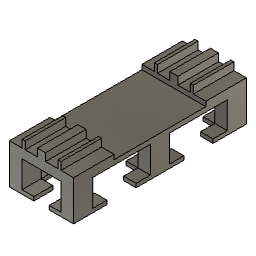
cell and oil channel flow sensors holder v5 kanishk fused v2 (Autodesk Fusion 360 design; units mm, degrees)
Autodesk Fusion 360 part; units mm, degrees
note: some values were not read from the file. Chosen so that the rebuilt part matches the saved one: which bodies a step acts on; which face or edge a step refers to.
sketch "Sketch1" plane through (0, 0, 0) normal (0, 0, 1) x (1, 0, 0)
  line L0 (0, 0) -> (86.6, 0)
  line L1 (86.6, 0) -> (86.6, 120)
  line L2 (86.6, 120) -> (0, 120)
  line L3 (0, 120) -> (0, 0)
  line L4 (43.3, 120) -> (35, 120)
  line L5 (35, 120) -> (35, 0)
  line L6 (35, 0) -> (43.3, 0)
  line L7 (43.3, 0) -> (43.3, 120)
  line L8 (43.3, 120) -> (51.6, 120)
  line L9 (51.6, 120) -> (51.6, 0)
  line L10 (51.6, 0) -> (43.3, 0)
  line L11 (43.3, 0) -> (43.3, 120)
  line L12 (51.6, 120) -> (66.2, 120)
  line L13 (66.2, 120) -> (66.2, 0)
  line L14 (66.2, 0) -> (51.6, 0)
  line L15 (51.6, 0) -> (51.6, 120)
  line L16 (66.2, 120) -> (70.2, 120)
  line L17 (70.2, 120) -> (70.2, 0)
  line L18 (70.2, 0) -> (66.2, 0)
  line L19 (66.2, 0) -> (66.2, 120)
  line L20 (70.2, 120) -> (84.8, 120)
  line L21 (84.8, 120) -> (84.8, 0)
  line L22 (84.8, 0) -> (70.2, 0)
  line L23 (70.2, 0) -> (70.2, 120)
  line L24 (84.8, 120) -> (90.8, 120)
  line L25 (90.8, 120) -> (90.8, 0)
  line L26 (90.8, 0) -> (84.8, 0)
  line L27 (84.8, 0) -> (84.8, 120)
  line L28 (35, 120) -> (20.4, 120)
  line L29 (20.4, 120) -> (20.4, 0)
  line L30 (20.4, 0) -> (35, 0)
  line L31 (35, 0) -> (35, 120)
  line L32 (20.4, 120) -> (16.4, 120)
  line L33 (16.4, 120) -> (16.4, 0)
  line L34 (16.4, 0) -> (20.4, 0)
  line L35 (20.4, 0) -> (20.4, 120)
  line L36 (16.4, 120) -> (1.8, 120)
  line L37 (1.8, 120) -> (1.8, 0)
  line L38 (1.8, 0) -> (16.4, 0)
  line L39 (16.4, 0) -> (16.4, 120)
  line L40 (1.8, 120) -> (-4.2, 120)
  line L41 (-4.2, 120) -> (-4.2, 0)
  line L42 (-4.2, 0) -> (1.8, 0)
  line L43 (1.8, 0) -> (1.8, 120)
  dimension "d1" = 86.6
  dimension "d2" = 120
  dimension "d3" = 8.3
  dimension "d4" = 120
  dimension "d5" = 8.3
  dimension "d6" = 120
  dimension "d7" = 14.6
  dimension "d8" = 120
  dimension "d9" = 4
  dimension "d10" = 120
  dimension "d11" = 14.6
  dimension "d12" = 120
  dimension "d13" = 6
  dimension "d14" = 14.6
  dimension "d15" = 120
  dimension "d16" = 4
  dimension "d17" = 120
  dimension "d18" = 14.6
  dimension "d19" = 120
  dimension "d20" = 6
  dimension "d21" = 120
  constraint horizontal L0
  constraint vertical L1
  constraint horizontal L2
  constraint vertical L3
  constraint coincident L0.start L3.end
  constraint horizontal L4
  constraint vertical L5
  constraint horizontal L6
  constraint vertical L7
  constraint midpoint L2 L4.start
  constraint horizontal L8
  constraint vertical L9
  constraint horizontal L10
  constraint vertical L11
  constraint horizontal L12
  constraint vertical L13
  constraint horizontal L14
  constraint vertical L15
  constraint horizontal L16
  constraint vertical L17
  constraint horizontal L18
  constraint vertical L19
  constraint horizontal L20
  constraint vertical L21
  constraint horizontal L22
  constraint vertical L23
  constraint horizontal L24
  constraint vertical L25
  constraint horizontal L26
  constraint vertical L27
  constraint horizontal L28
  constraint vertical L29
  constraint horizontal L30
  constraint vertical L31
  constraint horizontal L32
  constraint vertical L33
  constraint horizontal L34
  constraint vertical L35
  constraint horizontal L36
  constraint vertical L37
  constraint horizontal L38
  constraint vertical L39
  constraint horizontal L40
  constraint vertical L41
  constraint horizontal L42
  constraint vertical L43
  measures "d1" distance of L0.start L0.end
  measures "d2" distance of L0.start L2.end
  measures "d3" distance of L4.start L4.end
  measures "d4" distance of L4.start L6.end
  measures "d5" distance of L4.start L8.end
  measures "d6" distance of L4.start L6.end
  measures "d7" distance of L8.end L12.end
  measures "d8" distance of L8.end L9.end
  measures "d9" distance of L12.end L16.end
  measures "d10" distance of L12.end L13.end
  measures "d11" distance of L16.end L20.end
  measures "d12" distance of L16.end L17.end
  measures "d13" distance of L20.end L24.end
  measures "d14" distance of L4.end L28.end
  measures "d15" distance of L4.end L5.end
  measures "d16" distance of L28.end L32.end
  measures "d17" distance of L28.end L29.end
  measures "d18" distance of L32.end L36.end
  measures "d19" distance of L32.end L33.end
  measures "d20" distance of L36.end L40.end
  measures "d21" distance of L36.end L37.end
extrude "Extrude1" add sketch "Sketch1" along normal blind 52.3 contours L0 L2 L3 L37 L40 L42 L43 | L0 L2 L33 L36 L37 L38 L39 L43 | L0 L2 L29 L32 L33 L34 L35 L39 | L0 L2 L5 L28 L29 L30 L31 L35 | L0 L2 L4 L5 L6 L7 L11 L31 | L0 L2 L7 L8 L9 L10 L11 L15 | L0 L2 L9 L12 L13 L14 L15 L19 | L0 L2 L13 L16 L17 L18 L19 L23 | L0 L2 L17 L20 L21 L22 L23 L27 | L0 L1 L2 L21 L24 L26 L27 makes body 1
extrude "Extrude2" add sketch "Sketch1" along normal blind 62.3 contours L0 L2 L4 L5 L6 L7 L11 L31 | L0 L2 L7 L8 L9 L10 L11 L15 bodies 1
extrude "Extrude3" add sketch "Sketch1" along normal blind 62.3 contours L0 L2 L3 L37 L40 L42 L43 | L3 L40 L41 L42 | L0 L2 L29 L32 L33 L34 L35 L39 | L0 L2 L13 L16 L17 L18 L19 L23 | L0 L1 L2 L21 L24 L26 L27 | L1 L24 L25 L26 bodies 1
extrude "Extrude4" cut sketch "Sketch1" along normal blind 37.3 contours L3 L40 L41 L42 | L1 L24 L25 L26 bodies 1
sketch "Sketch2" plane through (0, 0, 0) normal (0, -1, 0) x (1, 0, 0)
  line L0 (86.6, 37.3) -> (90.8, 37.3)
  line L1 (90.8, 37.3) -> (90.8, 62.3)
  line L2 (90.8, 62.3) -> (84.8, 62.3)
  line L3 (84.8, 62.3) -> (84.8, 52.3)
  line L4 (84.8, 52.3) -> (70.2, 52.3)
  line L5 (70.2, 52.3) -> (70.2, 62.3)
  line L6 (70.2, 62.3) -> (66.2, 62.3)
  line L7 (66.2, 62.3) -> (66.2, 52.3)
  line L8 (66.2, 52.3) -> (51.6, 52.3)
  line L9 (51.6, 52.3) -> (51.6, 62.3)
  line L10 (51.6, 62.3) -> (35, 62.3)
  line L11 (35, 62.3) -> (35, 52.3)
  line L12 (35, 52.3) -> (20.4, 52.3)
  line L13 (20.4, 52.3) -> (20.4, 62.3)
  line L14 (20.4, 62.3) -> (16.4, 62.3)
  line L15 (16.4, 62.3) -> (16.4, 52.3)
  line L16 (16.4, 52.3) -> (1.8, 52.3)
  line L17 (1.8, 52.3) -> (1.8, 62.3)
  line L18 (1.8, 62.3) -> (-4.2, 62.3)
  line L19 (-4.2, 62.3) -> (-4.2, 37.3)
  line L20 (-4.2, 37.3) -> (0, 37.3)
  line L21 (0, 37.3) -> (0, 0)
  line L22 (0, 0) -> (86.6, 0)
  line L23 (86.6, 0) -> (86.6, 37.3)
  line L24 (0, 0) -> (10, 0)
  line L25 (10, 0) -> (10, 10)
  line L26 (10, 10) -> (0, 10)
  line L27 (0, 10) -> (0, 0)
  line L28 (86.6, 0) -> (76.6, 0)
  line L29 (76.6, 0) -> (76.6, 10)
  line L30 (76.6, 10) -> (86.6, 10)
  line L31 (86.6, 10) -> (86.6, 0)
  line L32 (0, 15) -> (10, 15)
  line L33 (10, 15) -> (10, 25)
  line L34 (10, 25) -> (0, 25)
  line L35 (0, 25) -> (0, 15)
  line L36 (0, 30) -> (10, 30)
  line L37 (10, 30) -> (10, 40)
  line L38 (10, 40) -> (0, 40)
  line L39 (0, 40) -> (0, 30)
  line L40 (86.6, 14.8875) -> (76.6, 14.8875)
  line L41 (76.6, 14.8875) -> (76.6, 24.8875)
  line L42 (76.6, 24.8875) -> (86.6, 24.8875)
  line L43 (86.6, 24.8875) -> (86.6, 14.8875)
  line L44 (86.6, 30.0734) -> (76.6, 30.0734)
  line L45 (76.6, 30.0734) -> (76.6, 40.0734)
  line L46 (76.6, 40.0734) -> (86.6, 40.0734)
  line L47 (86.6, 40.0734) -> (86.6, 30.0734)
  dimension "d30" = 10
  dimension "d31" = 10
  dimension "d32" = 10
  dimension "d33" = 10
  dimension "d34" = 10
  dimension "d35" = 10
  dimension "d36" = 10
  dimension "d37" = 10
  dimension "d38" = 10
  dimension "d39" = 10
  dimension "d40" = 10
  dimension "d41" = 10
  constraint horizontal L24
  constraint vertical L25
  constraint horizontal L26
  constraint vertical L27
  constraint coincident L21.end L22.start
  constraint horizontal L28
  constraint vertical L29
  constraint horizontal L30
  constraint vertical L31
  constraint coincident L22.end L23.start
  constraint horizontal L32
  constraint vertical L33
  constraint horizontal L34
  constraint vertical L35
  constraint coincident L21 L32.start
  constraint horizontal L36
  constraint vertical L37
  constraint horizontal L38
  constraint vertical L39
  constraint coincident L21 L36.start
  constraint horizontal L40
  constraint vertical L41
  constraint horizontal L42
  constraint vertical L43
  constraint coincident L23 L40.start
  constraint horizontal L44
  constraint vertical L45
  constraint horizontal L46
  constraint vertical L47
  constraint coincident L23 L44.start
  measures "d30" distance of L21.end L24.end
  measures "d31" distance of L21.end L26.end
  measures "d32" distance of L22.end L28.end
  measures "d33" distance of L22.end L30.end
  measures "d34" distance of L32.start L32.end
  measures "d35" distance of L32.start L34.end
  measures "d36" distance of L36.start L36.end
  measures "d37" distance of L36.start L38.end
  measures "d38" distance of L40.start L40.end
  measures "d39" distance of L40.start L42.end
  measures "d40" distance of L44.start L44.end
  measures "d41" distance of L44.start L46.end
extrude "Extrude5" cut sketch "Sketch2" against normal blind 20 contours L21 L22 L24 L25 L26 L27 bodies 1
extrude "Extrude6" add sketch "Sketch2" along normal blind 20 contours L22 L23 L28 L29 L30 L31 bodies 1
extrude "Extrude7" add sketch "Sketch2" along normal blind 20 contours L21 L32 L33 L34 L35 bodies 1
extrude "Extrude8" cut sketch "Sketch2" against normal blind 20 contours L23 L40 L41 L42 L43 bodies 1
extrude "Extrude9" cut sketch "Sketch2" against normal blind 20 contours L21 L36 L37 L38 L39 bodies 1
extrude "Extrude10" add sketch "Sketch2" along normal blind 20 contours L23 L44 L45 L46 L47 bodies 1
sketch "Sketch3" plane through (0, 0, 0) normal (0, -1, 0) x (1, 0, 0)
  line L0 (0, 0) -> (86.5609, 0)
  line L1 (43.2804, 0) -> (16.2804, 0)
  line L2 (16.2804, 0) -> (16.2804, 40)
  line L3 (16.2804, 40) -> (43.2804, 40)
  line L4 (43.2804, 40) -> (43.2804, 0)
  line L5 (43.2804, 0) -> (70.2804, 0)
  line L6 (70.2804, 0) -> (70.2804, 40)
  line L7 (70.2804, 40) -> (43.2804, 40)
  line L8 (43.2804, 40) -> (43.2804, 0)
  dimension "d54" = 27
  dimension "d55" = 40
  dimension "d56" = 27
  dimension "d57" = 40
  constraint coincident L0.start origin
  constraint horizontal L0
  constraint horizontal L1
  constraint vertical L2
  constraint horizontal L3
  constraint vertical L4
  constraint midpoint L0 L1.start
  constraint horizontal L5
  constraint vertical L6
  constraint horizontal L7
  constraint vertical L8
  measures "d54" distance of L1.start L1.end
  measures "d55" distance of L1.start L3.end
  measures "d56" distance of L1.start L5.end
  measures "d57" distance of L1.start L3.end
sketch "Sketch4" plane through (86.6, 0, 0) normal (1, 0, 0) x (0, 1, 0)
  line L0 (0, 24.8875) -> (20, 24.8875)
  line L1 (20, 24.8875) -> (20, 14.8875)
  line L2 (20, 14.8875) -> (0, 14.8875)
  line L3 (0, 14.8875) -> (0, 10)
  line L4 (0, 10) -> (-20, 10)
  line L5 (-20, 10) -> (-20, 0)
  line L6 (-20, 0) -> (120, 0)
  line L7 (120, 0) -> (120, 37.3)
  line L8 (120, 37.3) -> (0, 37.3)
  line L9 (0, 37.3) -> (0, 40.0734)
  line L10 (0, 40.0734) -> (-20, 40.0734)
  line L11 (-20, 40.0734) -> (-20, 30.0734)
  line L12 (-20, 30.0734) -> (0, 30.0734)
  line L13 (0, 30.0734) -> (0, 24.8875)
  line L14 (30, 0) -> (100, 0)
  line L15 (100, 0) -> (100, 35)
  line L16 (100, 35) -> (30, 35)
  line L17 (30, 35) -> (30, 0)
  dimension "d58" = 70
  dimension "d59" = 35
  constraint horizontal L14
  constraint vertical L15
  constraint horizontal L16
  constraint vertical L17
  constraint coincident L6 L14.start
  measures "d58" distance of L14.start L14.end
  measures "d59" distance of L14.start L16.end
extrude "Extrude11" cut sketch "Sketch3" against normal blind 130 bodies 1
extrude "Extrude12" cut sketch "Sketch4" against normal blind 100 contours L6 L14 L15 L16 L17 bodies 1
sketch "Sketch5" plane through (0, 0, 0) normal (0, -1, 0) x (1, 0, 0)
sketch "Sketch6" plane through (0, 0, 62.3) normal (0, 0, 1) x (-1, 0, 0)
  line L0 (-84.8, 0) -> (-90.8, 0)
  line L1 (-90.8, 0) -> (-90.8, -120)
  line L2 (-90.8, -120) -> (-84.8, -120)
  line L3 (-84.8, -120) -> (-84.8, 0)
  line L4 (-84.8, 0) -> (-86.3, 0)
  line L5 (-86.3, 0) -> (-86.3, -120)
  line L6 (-86.3, -120) -> (-84.8, -120)
  line L7 (-84.8, -120) -> (-84.8, 0)
  dimension "d64" = 1.5
  dimension "d65" = 120
  constraint horizontal L4
  constraint vertical L5
  constraint horizontal L6
  constraint vertical L7
  constraint coincident L0.start L3.end
  measures "d64" distance of L0.start L4.end
  measures "d65" distance of L0.start L2.end
sketch "Sketch7" plane through (0, 0, 62.3) normal (0, 0, 1) x (-1, 0, 0)
  line L0 (-1.8, 0) -> (-1.8, -120)
  line L1 (-1.8, -120) -> (4.2, -120)
  line L2 (4.2, -120) -> (4.2, 0)
  line L3 (4.2, 0) -> (-1.8, 0)
  line L4 (-1.8, -120) -> (-0.3, -120)
  line L5 (-0.3, -120) -> (-0.3, 0)
  line L6 (-0.3, 0) -> (-1.8, 0)
  line L7 (-1.8, 0) -> (-1.8, -120)
  dimension "d66" = 1.5
  dimension "d67" = 120
  constraint horizontal L4
  constraint vertical L5
  constraint horizontal L6
  constraint vertical L7
  constraint coincident L0.end L1.start
  measures "d66" distance of L0.end L4.end
  measures "d67" distance of L0.end L0.start
extrude "Extrude13" cut sketch "Sketch6" sketch "Sketch7" against normal blind 10 contours L0 L2 L3 L4 L5 L6 L7 of sketch 2 contours L0 L1 L3 L4 L5 L6 L7 bodies 1
sketch "Sketch8" plane through (0, 0, 62.3) normal (0, 0, 1) x (-1, 0, 0)
  line L0 (-51.6, 0) -> (-51.6, -120)
  line L1 (-51.6, -120) -> (-35, -120)
  line L2 (-35, -120) -> (-35, 0)
  line L3 (-35, 0) -> (-51.6, 0)
  line L4 (-35, -120) -> (-36.5, -120)
  line L5 (-36.5, -120) -> (-36.5, 0)
  line L6 (-36.5, 0) -> (-35, 0)
  line L7 (-35, 0) -> (-35, -120)
  line L8 (-51.6, -120) -> (-50.1, -120)
  line L9 (-50.1, -120) -> (-50.1, 0)
  line L10 (-50.1, 0) -> (-51.6, 0)
  line L11 (-51.6, 0) -> (-51.6, -120)
  dimension "d70" = 1.5
  dimension "d71" = 120
  dimension "d72" = 1.5
  dimension "d73" = 120
  constraint horizontal L4
  constraint vertical L5
  constraint horizontal L6
  constraint vertical L7
  constraint coincident L1.end L2.start
  constraint horizontal L8
  constraint vertical L9
  constraint horizontal L10
  constraint vertical L11
  constraint coincident L0.end L1.start
  measures "d70" distance of L1.end L4.end
  measures "d71" distance of L1.end L2.end
  measures "d72" distance of L0.end L8.end
  measures "d73" distance of L0.end L0.start
extrude "Extrude14" cut sketch "Sketch8" against normal blind 10 contours L0 L1 L3 L8 L9 L10 L11 | L1 L2 L3 L4 L5 L6 L7 bodies 1
extrude "Extrude15" cut sketch "Sketch1" along normal blind 100 contours L3 L40 L41 L42 | L1 L24 L25 L26 bodies 1
extrude "Extrude16" cut 1 faces at (86.4, 80, 62.3) along direction (0, 0, -1) blind 10 on bodies 1 bodies 1
extrude "Extrude17" cut 1 faces at (0.1, 80, 62.3) along direction (0, 0, -1) blind 10 on bodies 1 bodies 1
sketch "Sketch9" plane through (0, 0, 0) normal (0, -1, 0) x (1, 0, 0)
extrude "Extrude18" cut 3 faces at (3.3333, -20, 21.6667) (83.2667, -20, 33.4067) (83.2667, -20, 3.3333) along direction (0, 1, 0) blind 20 on bodies 1 bodies 1
extrude "Extrude19" add 1 faces at (76.6, 6.6667, 18.2208) along direction (1, 0, 0) blind 10 on bodies 1 bodies 1
extrude "Extrude20" add 2 faces at (3.3333, 20, 36.6667) (6.6667, 20, 3.3333) along direction (0, -1, 0) blind 20 on bodies 1 bodies 1
mirror "Mirror1" about plane through (51.6, 120, 0) normal (0, 1, 0) of bodies 1 merged
extrude "Extrude21" cut 1 faces at (81.1601, 240, 30.7667) along direction (0, -1, 0) blind 5 on bodies 1 bodies 1
extrude "Extrude22" cut 1 faces at (81.1601, 0, 30.7667) along direction (0, 1, 0) blind 5 on bodies 1 bodies 1
split "Split1" by plane through (36.5, 120, 62.3) normal (-1, 0, 0) bodies 1 makes body 2 at (0, 126.6667, 11.6667)
extrude "Extrude23" cut 2 faces at (36.5, 81.6667, 48.2) (36.5, 158.3333, 58.9667) along direction (1, 0, 0) blind 3 on bodies 1 bodies 1
move_body "Move1" bodies 2 to x (1, 0, 0) y (0, 1, 0) z (0, 0, 1) at (3, 0, 0)
combine "Combine1" operation add target body 1 tool bodies 2
sketch "Sketch10" plane through (19.2804, 0, 0) normal (1, 0, 0) x (0, 1, 0)
  line L0 (5, 40) -> (5, 0)
  line L1 (5, 0) -> (30, 0)
  line L2 (30, 0) -> (30, 35)
  line L3 (30, 35) -> (100, 35)
  line L4 (100, 35) -> (100, 0)
  line L5 (100, 0) -> (140, 0)
  line L6 (140, 0) -> (140, 35)
  line L7 (140, 35) -> (210, 35)
  line L8 (210, 35) -> (210, 0)
  line L9 (210, 0) -> (235, 0)
  line L10 (235, 0) -> (235, 40)
  line L11 (235, 40) -> (5, 40)
  line L12 (5, 0) -> (30, 0)
  line L13 (30, 0) -> (30, 5)
  line L14 (30, 5) -> (5, 5)
  line L15 (5, 5) -> (5, 0)
  line L16 (100, 0) -> (140, 0)
  line L17 (140, 0) -> (140, 5)
  line L18 (140, 5) -> (100, 5)
  line L19 (100, 5) -> (100, 0)
  line L20 (210, 0) -> (235, 0)
  line L21 (235, 0) -> (235, 5)
  line L22 (235, 5) -> (210, 5)
  line L23 (210, 5) -> (210, 0)
  line L24 (100, 35) -> (107.5, 35)
  line L25 (107.5, 35) -> (107.5, 0)
  line L26 (107.5, 0) -> (100, 0)
  line L27 (100, 0) -> (100, 35)
  line L28 (140, 0) -> (132.5, 0)
  line L29 (132.5, 0) -> (132.5, 35)
  line L30 (132.5, 35) -> (140, 35)
  line L31 (140, 35) -> (140, 0)
  dimension "d96" = 5
  dimension "d97" = 5
  dimension "d98" = 5
  dimension "d99" = 7.5
  dimension "d100" = 7.5
  dimension "d101" = 35
  constraint horizontal L12
  constraint vertical L13
  constraint horizontal L14
  constraint vertical L15
  constraint coincident L0.end L1.start
  constraint horizontal L16
  constraint vertical L17
  constraint horizontal L18
  constraint vertical L19
  constraint coincident L4.end L5.start
  constraint horizontal L20
  constraint vertical L21
  constraint horizontal L22
  constraint vertical L23
  constraint coincident L8.end L9.start
  constraint horizontal L24
  constraint vertical L25
  constraint horizontal L26
  constraint vertical L27
  constraint coincident L3.end L4.start
  constraint horizontal L28
  constraint vertical L29
  constraint horizontal L30
  constraint vertical L31
  constraint coincident L5.end L6.start
  measures "d96" distance of L0.end L14.end
  measures "d97" distance of L4.end L18.end
  measures "d98" distance of L8.end L22.end
  measures "d99" distance of L3.end L24.end
  measures "d100" distance of L5.end L28.end
  measures "d101" distance of L5.end L6.end
extrude "Extrude24" add sketch "Sketch10" along normal blind 51 contours L0 L1 L2 L12 L13 L14 L15 | L8 L9 L10 L20 L21 L22 L23 | L4 L5 L16 L18 L19 L25 L26 L27 | L5 L16 L18 L25 L29 | L5 L6 L16 L17 L18 L28 L29 L31 bodies 1
extrude "Extrude25" cut sketch "Sketch10" along normal blind 1000 and the other way blind 100 contours L4 L18 L24 L25 L27 | L4 L5 L16 L18 L19 L25 L26 L27 | L6 L18 L29 L30 L31 | L5 L6 L16 L17 L18 L28 L29 L31 bodies 1
sketch "Sketch12" plane through (0, 235, 0) normal (0, 1, 0) x (-1, 0, 0)
  line L0 (-86.6, 0) -> (-3, 0)
  line L1 (-3, 0) -> (-3, 52.3)
  line L2 (-3, 52.3) -> (-19.4, 52.3)
  line L3 (-19.4, 52.3) -> (-19.4, 62.3)
  line L4 (-19.4, 62.3) -> (-23.4, 62.3)
  line L5 (-23.4, 62.3) -> (-23.4, 52.3)
  line L6 (-23.4, 52.3) -> (-39.5, 52.3)
  line L7 (-39.5, 52.3) -> (-39.5, 62.3)
  line L8 (-39.5, 62.3) -> (-50.1, 62.3)
  line L9 (-50.1, 62.3) -> (-50.1, 52.3)
  line L10 (-50.1, 52.3) -> (-66.2, 52.3)
  line L11 (-66.2, 52.3) -> (-66.2, 62.3)
  line L12 (-66.2, 62.3) -> (-70.2, 62.3)
  line L13 (-70.2, 62.3) -> (-70.2, 52.3)
  line L14 (-70.2, 52.3) -> (-86.6, 52.3)
  line L15 (-86.6, 52.3) -> (-86.6, 0)
  line L16 (-19.2804, 5) -> (-70.2804, 5)
  line L17 (-70.2804, 5) -> (-70.2804, 40)
  line L18 (-70.2804, 40) -> (-19.2804, 40)
  line L19 (-19.2804, 40) -> (-19.2804, 5)
  line L20 (-70.2804, 5) -> (-86.6, 5)
  line L21 (-86.6, 5) -> (-86.6, 0)
  line L22 (-86.6, 0) -> (-70.2804, 0)
  line L23 (-70.2804, 0) -> (-70.2804, 5)
  line L24 (-19.2804, 5) -> (-3, 5)
  line L25 (-3, 5) -> (-3, 0)
  line L26 (-3, 0) -> (-19.2804, 0)
  line L27 (-19.2804, 0) -> (-19.2804, 5)
  line L28 (-44.8, 0) -> (-54.8, 0)
  line L29 (-54.8, 0) -> (-54.8, 5)
  line L30 (-54.8, 5) -> (-44.8, 5)
  line L31 (-44.8, 5) -> (-44.8, 0)
  line L32 (-34.8, 0) -> (-34.8, 5)
  dimension "d108" = 10
  constraint horizontal L20
  constraint vertical L21
  constraint horizontal L22
  constraint vertical L23
  constraint coincident L0.start L15.end
  constraint coincident L16.end L17.start
  constraint horizontal L24
  constraint vertical L25
  constraint horizontal L26
  constraint vertical L27
  constraint coincident L0.end L1.start
  constraint coincident L16.start L19.end
  constraint horizontal L28
  constraint vertical L29
  constraint horizontal L30
  constraint vertical L31
  constraint midpoint L0 L28.start
  constraint symmetric L28.end L31 L32.start
  constraint symmetric L29.end L31 L32.end
  measures "d108" distance of L28.start L28.end
extrude "Extrude26" cut sketch "Sketch12" against normal blind 1000 contours L0 L16 L28 L29 L30 L31 | L0 L16 L31 L32 bodies 1
extrude "Extrude27" add sketch "Sketch12" against normal blind 205 contours L0 L15 L20 L21 L22 L23 | L0 L1 L24 L25 L26 L27 bodies 1
sketch "Sketch13" plane through (3, 0, 0) normal (-1, 0, 0) x (0, -1, 0)
  line L0 (-210, 5) -> (-210, 35)
  line L1 (-210, 35) -> (-132.5, 35)
  line L2 (-132.5, 35) -> (-132.5, 5)
  line L3 (-132.5, 5) -> (-210, 5)
  line L4 (-107.5, 5) -> (-107.5, 35)
  line L5 (-107.5, 35) -> (-30, 35)
  line L6 (-30, 35) -> (-30, 5)
  line L7 (-30, 5) -> (-107.5, 5)
  line L8 (-235, 0) -> (-5, 0)
  line L9 (-5, 0) -> (-5, 52.3)
  line L10 (-5, 52.3) -> (-235, 52.3)
  line L11 (-235, 52.3) -> (-235, 0)
  line L12 (-210, 5) -> (-132.5, 5)
  line L13 (-171.25, 5) -> (-191.25, 5)
  line L14 (-191.25, 5) -> (-191.25, 0)
  line L15 (-191.25, 0) -> (-171.25, 0)
  line L16 (-171.25, 0) -> (-171.25, 5)
  line L17 (-132.5, 5) -> (-107.5, 5)
  line L18 (-120, 5) -> (-120, 0)
  line L19 (-151.25, 5) -> (-151.25, 0)
  line L20 (-48.75, 5) -> (-48.75, 0)
  line L21 (-88.75, 5) -> (-88.75, 0)
  dimension "d113" = 20
  constraint coincident L0.start L3.end
  constraint coincident L2.end L3.start
  constraint horizontal L13
  constraint vertical L14
  constraint horizontal L15
  constraint vertical L16
  constraint midpoint L12 L13.start
  constraint coincident L4.start L7.end
  constraint midpoint L17 L18.start
  constraint midpoint L8 L18.end
  constraint symmetric L13.end L16 L19.start
  constraint symmetric L14.end L16 L19.end
  constraint symmetric L13.end L18 L20.start
  constraint symmetric L14.end L18 L20.end
  constraint symmetric L18 L19.start L21.start
  constraint symmetric L18 L19.end L21.end
  measures "d113" distance of L13.start L13.end
extrude "Extrude28" cut sketch "Sketch13" against normal blind 83.6 contours L3 L8 L12 L13 L14 L15 L16 | L3 L8 L12 L16 L19 | L7 L8 L20 L21 bodies 1
ref_plane "WorkPlane1" through (78.4, 120, 46.15) normal (0, 0, 1) x (1, 0, 0)
split "Split2" by plane through (78.4, 120, 46.15) normal (0, 0, 1) bodies 1 makes body 3 at (13.9333, 81.6667, 52.3)
move_body "Move2" bodies 1 to x (1, 0, 0) y (0, 1, 0) z (0, 0, 1) at (0, 0, -25)
extrude "Extrude29" cut 4 faces at (75.7203, 158.3333, 10) (81.1601, 81.6667, 10) (8.4268, 158.3333, 10) (8.4268, 55.8333, 10) along direction (0, 0, 1) blind 5 on bodies 1 bodies 1
ref_plane "WorkPlane2" through (44.8, 120, 54.225) normal (0, -1, 0) x (0, 0, -1)
split "Split3" by plane through (44.8, 120, 54.225) normal (0, -1, 0) bodies 3 makes body 4 at (30.8667, 43.3333, 46.15)
extrude "Extrude30" cut 1 faces at (46.5667, 120, 48.2) along direction (0, -1, 0) blind 50 on bodies 4 bodies 4
extrude "Extrude31" cut 1 faces at (46.5667, 120, 48.2) along direction (0, 1, 0) blind 50 on bodies 3 bodies 3
ref_plane "WorkPlane3" through (11.1402, 120, -2.5) normal (0, -1, 0) x (0, 0, -1)
split "Split4" by plane through (11.1402, 120, -2.5) normal (0, -1, 0) bodies 1 makes body 5 at (30.8667, 43.3333, 21.15)
move_body "Move3" bodies 1 to x (1, 0, 0) y (0, 1, 0) z (0, 0, 1) at (0, 10, 0)
move_body "Move4" bodies 5 to x (1, 0, 0) y (0, 1, 0) z (0, 0, 1) at (0, -10, 0)
split "Split5" by plane through (19.2804, -10, 15) normal (0, 0, -1) bodies 1 5 makes body 10 at (70.5601, 3.3333, -25) makes body 11 at (81.1601, 110, -10) makes body 12 at (8.4268, 110, -10) makes body 13 at (19.0268, 3.3333, -25) makes body 6 at (8.4268, 130, -10) makes body 7 at (70.5601, 236.6667, -25) makes body 8 at (19.0268, 236.6667, -25) makes body 9 at (81.1601, 130, -10)
move_body "Move5" bodies 12 11 to x (1, 0, 0) y (0, 1, 0) z (0, 0, 1) at (0, 10, 0)
move_body "Move6" bodies 6 9 to x (1, 0, 0) y (0, 1, 0) z (0, 0, 1) at (0, -10, 0)
extrude "Extrude32" add 1 faces at (36.2935, 130, 19.1) along direction (0, -1, 0) blind 20 on bodies 1 bodies 1 10 13 5 6 9 11 12
combine "Combine2" operation add target body 8 tool bodies 7 1 13 10
move_body "Move7" bodies 3 to x (1, 0, 0) y (0, 1, 0) z (0, 0, 1) at (0, 10, 0)
move_body "Move8" bodies 4 to x (1, 0, 0) y (0, 1, 0) z (0, 0, 1) at (0, -10, 0)
sketch "Sketch14" plane through (0, 0, 52.3) normal (0, 0, 1) x (-1, 0, 0)
  line L0 (-86.6, -60) -> (-70.2, -60)
  line L1 (-70.2, -60) -> (-70.2, 5)
  line L2 (-70.2, 5) -> (-86.6, 5)
  line L3 (-86.6, 5) -> (-86.6, -60)
  line L4 (-78.4, 5) -> (-78.4, 0)
  circle A0 centre (-78.4, 0) radius 2
  line L5 (-86.6, -27.5) -> (-69.3228, -27.5)
  circle A1 centre (-78.4, -55) radius 2
  line L6 (-78.4, -60) -> (-78.4, -55)
  line L7 (-3, 5) -> (-86.6, 5)
  line L8 (-44.8, 5) -> (-44.8, -64.8479)
  circle A2 centre (-11.2, -55) radius 2
  circle A3 centre (-11.2, 0) radius 2
  line L9 (-11.2, -60) -> (-11.2, -55)
  line L10 (-3, -27.5) -> (-20.2772, -27.5)
  line L11 (-11.2, 5) -> (-11.2, 0)
  line L12 (-86.6, 5) -> (-86.6, -245)
  line L13 (-86.6, -120) -> (15, -120)
  circle A4 centre (-78.4, -185) radius 2
  circle A5 centre (-11.2, -185) radius 2
  line L14 (-11.2, -180) -> (-11.2, -185)
  line L15 (-78.4, -180) -> (-78.4, -185)
  line L16 (-44.8, -245) -> (-44.8, -175.1521)
  line L17 (-3, -212.5) -> (-20.2772, -212.5)
  line L18 (-86.6, -212.5) -> (-69.3228, -212.5)
  circle A6 centre (-11.2, -240) radius 2
  line L19 (-11.2, -245) -> (-11.2, -240)
  circle A7 centre (-78.4, -240) radius 2
  line L20 (-78.4, -245) -> (-78.4, -240)
  line L21 (-86.6, -120) -> (-86.6, -7.5)
  line L22 (-86.6, -7.5) -> (6.5947, -7.5)
  line L23 (-86.6, -232.5) -> (6.5947, -232.5)
  circle A8 centre (-78.4, 0) radius 4
  circle A9 centre (-78.4, -55) radius 4
  circle A10 centre (-11.2, 0) radius 4
  circle A11 centre (-11.2, -55) radius 4
  circle A12 centre (-78.4, -240) radius 4
  circle A13 centre (-11.2, -240) radius 4
  circle A14 centre (-78.4, -185) radius 4
  circle A15 centre (-11.2, -185) radius 4
  dimension "d127" = 4
  dimension "d128" = 112.5
  dimension "d129" = 8
  constraint midpoint L2 L4.start
  constraint perpendicular L2 L4
  constraint coincident L4.end A0.centre
  constraint midpoint L3 L5.start
  constraint perpendicular L1 L5
  constraint symmetric L4.start L5 L6.start
  constraint symmetric L4.end L5 A1.centre
  constraint symmetric A0 L5 A1
  constraint coincident L2.end L3.start
  constraint midpoint L7 L8.start
  constraint perpendicular L7 L8
  constraint symmetric L4.start L8 L11.start
  constraint symmetric L4.end L8 A3.centre
  constraint symmetric A0 L8 A3
  constraint symmetric L5.start L8 L10.start
  constraint symmetric L5.end L8 L10.end
  constraint symmetric A1 L8 A2
  constraint symmetric L6.start L8 L9.start
  constraint symmetric A1.centre L8 A2.centre
  constraint perpendicular L2 L12
  constraint midpoint L12 L13.start
  constraint perpendicular L12 L13
  constraint symmetric L4.start L13 L20.start
  constraint symmetric L4.end L13 A7.centre
  constraint symmetric A0 L13 A7
  constraint symmetric L5.start L13 L18.start
  constraint symmetric L5.end L13 L18.end
  constraint symmetric A1 L13 A4
  constraint symmetric L6.start L13 L15.start
  constraint symmetric A1.centre L13 A4.centre
  constraint symmetric L8.start L13 L16.start
  constraint symmetric L8.end L13 L16.end
  constraint symmetric A2 L13 A5
  constraint symmetric A3 L13 A6
  constraint symmetric L9.start L13 L14.start
  constraint symmetric A2.centre L13 A5.centre
  constraint symmetric L10.start L13 L17.start
  constraint symmetric L10.end L13 L17.end
  constraint symmetric L11.start L13 L19.start
  constraint symmetric A3.centre L13 A6.centre
  constraint perpendicular L13 L21
  constraint perpendicular L8 L22
  constraint symmetric L13 L21.end L23.start
  constraint symmetric L13 L22.end L23.end
  constraint concentric A0 A8
  constraint symmetric L5 A8 A9
  constraint symmetric L8 A8 A10
  constraint symmetric L8 A9 A11
  constraint symmetric L13 A8 A12
  constraint symmetric L13 A9 A14
  constraint symmetric L13 A10 A13
  constraint symmetric L13 A11 A15
  measures "d127" diameter of A0
  measures "d128" distance of L13.start L21.end
  measures "d129" diameter of A8
extrude "Extrude33" cut sketch "Sketch14" against normal blind 77.3 contours A0 | A1 | A2 | A3 | A4 | A5 | A6 | A7 bodies 3 4 8
split "Split6" by plane through (19.2804, -10, 15) normal (0, 0, -1) bodies 8 makes body 14 at (8.4268, 115.8333, -25) makes body 15 at (86.6, 236.6667, -10) makes body 16 at (3, 3.3333, -10) makes body 17 at (86.6, 3.3333, -10) makes body 18 at (81.1601, 115.8333, -25) makes body 19 at (3, 236.6667, -10)
move_body "Move9" bodies 17 16 to x (1, 0, 0) y (0, 1, 0) z (0, 0, 1) at (0, 12, 0)
move_body "Move10" bodies 15 19 to x (1, 0, 0) y (0, 1, 0) z (0, 0, 1) at (0, -12, 0)
combine "Combine3" operation add target body 18 tool bodies 14 17 15 19 8 16
extrude "Extrude34" add 4 faces at (11.8592, 226.9937, 15) (10.7222, 11.6922, 15) (77.2521, 11.4472, 15) (77.9039, 227.4472, 15) along direction (0, 0, -1) blind 40 on bodies 18 bodies 18
move_body "Move11" bodies 4 to x (1, 0, 0) y (0, 1, 0) z (0, 0, 1) at (0, 0, -25)
move_body "Move12" bodies 3 to x (1, 0, 0) y (0, 1, 0) z (0, 0, 1) at (0, 0, -25)
combine "Combine4" operation add target body 18 tool bodies 3
combine "Combine5" operation add target body 4 tool bodies 18
extrude "Extrude35" cut 1 faces at (46.5667, -5, 19.1) along direction (0, 1, 0) blind 12 on bodies 4 bodies 4
extrude "Extrude36" cut 1 faces at (46.5667, 245, 19.1) along direction (0, -1, 0) blind 12 on bodies 4 bodies 4
extrude "Extrude37" add 1 faces at (46.5667, 60, 23.2) along direction (0, -1, 0) blind 10 on bodies 4 bodies 4
extrude "Extrude38" add 1 faces at (46.5667, 180, 23.2) along direction (0, 1, 0) blind 10 on bodies 4 bodies 4
extrude "Extrude39" add 4 faces at (77.5194, 185.4828, 21.15) (11.7749, 185.1186, 21.15) (79.1854, 55.4534, 21.15) (11.6887, 55.4534, 21.15) along direction (0, 0, -1) blind 6.15 on bodies 4 bodies 4
equation "d116 = ( -12.3 / 2 ) * 1 mm"
equation "d119 = ( -230 / 2 ) * 1 mm"
equation "d124 = ( -25 / 2 ) * 1 mm"
equation "d128 = ( 225 / 2 ) * 1 mm"
